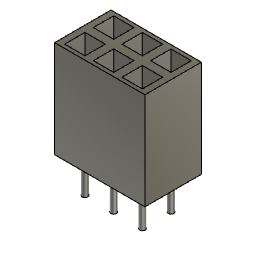
pinSocket_2.54mmp_2x3 (Autodesk Fusion 360 design; units mm, degrees)
Autodesk Fusion 360 part; units mm, degrees
sketch "スケッチ1" plane through (0, 0, 0) normal (0, 0, 1) x (1, 0, 0)
  line L0 (0, 0) -> (8, 0)
  line L1 (8, 0) -> (8, 5)
  line L2 (8, 5) -> (0, 5)
  line L3 (0, 5) -> (0, 0)
  circle A0 centre (1.46, 1.23) radius 0.25
  dimension "d1" = 8
  dimension "d2" = 5
  dimension "d15" = 0.5
  dimension "d16" = 1.23
  dimension "d17" = 1.46
  constraint horizontal L0
  constraint vertical L1
  constraint horizontal L2
  constraint vertical L3
  constraint coincident L0.start L3.end
  measures "d1" distance of L0.start L0.end
  measures "d2" distance of L0.start L2.end
  measures "d15" diameter of A0
  measures "d16" distance of L0 A0.centre
  measures "d17" distance of L3 A0.centre
extrude "押し出し1" add sketch "スケッチ1" along normal blind 8.6 contours L0 L1 L2 L3 | A0
sketch "スケッチ2" plane through (0, 0, 8.6) normal (0, 0, 1) x (-1, 0, 0)
  line L0 (0, -5) -> (0, 0)
  line L1 (0, 0) -> (-8, 0)
  line L2 (-8, 0) -> (-8, -5)
  line L3 (-8, -5) -> (0, -5)
  line L4 (-0.56, -0.33) -> (-2.36, -0.33)
  line L5 (-2.36, -0.33) -> (-2.36, -2.13)
  line L6 (-2.36, -2.13) -> (-0.56, -2.13)
  line L7 (-0.56, -2.13) -> (-0.56, -0.33)
  dimension "d5" = 1.8
  dimension "d6" = 1.8
  dimension "d7" = 0.33
  dimension "d8" = 0.56
  constraint horizontal L4
  constraint vertical L5
  constraint horizontal L6
  constraint vertical L7
  measures "d5" distance of L4.start L4.end
  measures "d6" distance of L4.start L6.end
  measures "d7" distance of L1 L4
  measures "d8" distance of L0 L7
extrude "押し出し2" cut sketch "スケッチ2" against normal blind 8 contours L4 L5 L6 L7
pattern_linear "R パターン1" count 3 spacing 2.54 along (1, 0, 0) count 2 spacing 2.54 along (0, 1, 0) of "押し出し2"
extrude "押し出し3" add sketch "スケッチ1" against normal blind 3 contours A0
pattern_linear "R パターン2" count 3 spacing 2.54 along (1, 0, 0) count 2 spacing 2.54 along (0, 1, 0) of "押し出し3"
